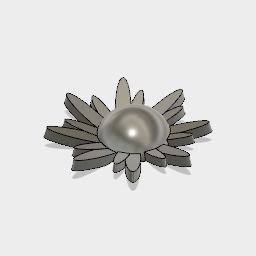
花 (Autodesk Fusion 360 design; units mm, degrees)
Autodesk Fusion 360 part; units mm, degrees
sketch "草图1" plane through (0, 0, 0) normal (0, 1, 0) x (1, 0, 0)
  ellipse E0 centre (0, 0) end of major axis (10, 0) minor radius 2
  line L0 (-10, 0) -> (10, 0)
  line L1 (0, -2) -> (0, 2)
  dimension "d1" = 4
extrude "拉伸1" add sketch "草图1" along normal blind 3 makes body 1
move_body "移动1" bodies 1 to x (0.965926, 0.258819, 0) y (-0.258819, 0.965926, 0) z (0, 0, 1) at (0, 0, 0)
sketch "草图3" plane through (0, 0, 0) normal (0, 0, 1) x (1, 0, 0)
sketch "草图4" plane through (0, 0, 0) normal (0, 1, 0) x (1, 0, 0)
box "长方体基本要素2" add length 2 width 2 height 2 placed x (0, 0, -1) y (-1, 0, 0) z (0, 1, 0) at (-13, 0, 0) separate body makes body 2
move_body "移动7" bodies 2 to x (1, 0, 0) y (0, 1, 0) z (0, 0, 1) at (0.9169, 0, 1.2607)
move_body "移动8" bodies 2 to x (1, 0, 0) y (0, 1, 0) z (0, 0, 1) at (0.1146, -2.0057, 0)
pattern_circular "C-阵列1" count 8 over 360 about axis through (-11.9685, -0.0057, 1.2607) along (0, -1, 0) of bodies 1 makes body 3 at (-1.3348, 0.645, 10.9573) makes body 4 at (-11.3059, 0.645, 15.6364) makes body 5 at (-21.6652, 0.645, 11.8944) makes body 6 at (-25.5678, 3.5428, 1.9233) makes body 7 at (-22.6022, 0.645, -8.4359) makes body 8 at (-12.6311, 0.645, -13.115) makes body 9 at (-2.2719, 0.645, -9.373)
copy_body "复制和粘贴实体1" bodies 9 3 1 6 7 8 5 4 makes body 10 makes body 11 makes body 12 makes body 13 makes body 14 makes body 15 makes body 16 makes body 17
scale "缩放1" factor 0.8 about (-13.2292, 0.3096, -0.2721) bodies 15 14 13 16 17 11 12 10
move_body "移动9" bodies 10 15 14 13 16 17 11 12 to x (0.965926, 0, 0.258819) y (0, 1, 0) z (-0.258819, 0, 0.965926) at (-0.0815, 0, 3.1406)
sphere "球体基本要素1" add diameter 20 placed x (1, 0, 0) y (0, 0, -1) z (0, 1, 0) at (-48, 0, 5) separate body makes body 18
move_body "MoveFace1" bodies 18 to x (1, 0, 0) y (0, 1, 0) z (0, 0, 1) at (36.2681, -1.0229, -5.7526) on bodies 18
combine "合并1" operation add target body 18 tool bodies 1 5 17 8 4 15 7 14 16 12 11 3 6 9 10 13
box "长方体基本要素4" add length 29.7479 width 64.589 height 20 placed x (0, 0, 1) y (1, 0, 0) z (0, 1, 0) at (27.6012, 0, -3.4705) separate body makes body 19
move_body "移动10" bodies 19 to x (1, 0, 0) y (0, -1, 0) z (0, 0, -1) at (-68.1059, -0.6046, 12.2656)
move_body "移动11" bodies 19 to x (1, 0, 0) y (0, 1, 0) z (0, 0, 1) at (0, 0.4248, 0)
combine "合并2" operation cut target body 18 tool bodies 19
hidden bodies 2
